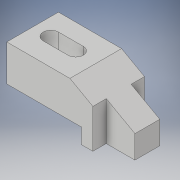
# Autodesk Inventor part: 410571040-T1
Saved by Autodesk Inventor 2017 (Build 210142000, 142)
## iProperties
Part Number: 410571040-T1
Material: 一般
Document SubType Name: Modeling
Designer: user
Density: 1 g/cm^3
Appearance: 預設
Author: user
Autodesk Inventor part; units mm, degrees
ref_plane "YZ Plane" through (0, 0, 0) normal (1, 0, 0) x (0, 1, 0)
ref_plane "XZ Plane" through (0, 0, 0) normal (0, 1, 0) x (-1, 0, 0)
ref_plane "XY Plane" through (0, 0, 0) normal (0, 0, 1) x (1, 0, 0)
sketch "草圖1" plane through (0, 0, 0) normal (0, 0, 1) x (1, 0, 0)
  line L0 (0, 0) -> (0, 38)
  line L1 (0, 38) -> (66, 38)
  line L2 (66, 38) -> (120, 8)
  line L3 (120, 8) -> (120, -16)
  line L4 (120, -16) -> (78, -16)
  line L5 (78, -16) -> (78, 0)
  line L6 (78, 0) -> (0, 0)
  dimension "d0" = 54
  dimension "d1" = 38
  dimension "d2" = 24
  dimension "d3" = 42
  dimension "d4" = 66
  dimension "d5" = 120
  constraints: 14 end point, 4 perpendicular, 1 parallel, 1 vertical
  measures "d0" distance between parallel lines of L4 L1
  measures "d1" distance of L0.start L0.end
  measures "d2" distance of L2.end L3.end
  measures "d3" distance of L3.end L4.end
  measures "d4" distance of L0.end L1.end
  measures "d5" distance between parallel lines of L3 L0
extrude "擠出1" add sketch "草圖1" against normal blind 54
sketch "草圖2" plane through (0, 38, 0) normal (0, 1, 0) x (1, 0, 0)
  arc A0 (18, 36) -> (18, 20) centre (18, 28) ccw
  line L0 (18, 36) -> (44, 36)
  line L1 (18, 20) -> (44, 20)
  arc A1 (44, 20) -> (44, 36) centre (44, 28) ccw
  line L2 (0, 0) -> (66, 0) projected
  line L3 (0, 0) -> (0, 54) projected
  dimension "d8" = 28
  dimension "d9" = 16
  dimension "d10" = 18
  dimension "d11" = 26
  constraints: 4 end point, 4 point on circle, 4 tangent, 2 centre point, 1 horizontal, 1 parallel
  measures "d8" distance from line of A0.centre L2
  measures "d9" distance between parallel lines of L1 L0
  measures "d10" distance from line of L3 A0.centre
  measures "d11" distance of A1.centre A0.centre
extrude "擠出2" cut sketch "草圖2" against normal up to next
sketch "草圖3" plane through (78, -16, 0) normal (0, -1, 0) x (1, 0, 0)
  line L0 (12, -54) -> (12, -40)
  line L1 (12, -40) -> (42, -40)
  line L2 (42, -40) -> (42, -54)
  line L3 (42, -54) -> (12, -54)
  line L4 (42, 0) -> (42, -54) projected
  line L5 (42, -27) -> (-15.5842, -27)
  line L6 (12, 0) -> (12, -14)
  line L7 (12, -14) -> (42, -14)
  line L8 (42, -14) -> (42, 0)
  line L9 (42, 0) -> (12, 0)
  line L10 (42, -54) -> (42, 0)
  point P0 (-78, 0)
  point P1 (0, 0)
  point P2 (0, -54)
  point P3 (0, 0)
  dimension "d18" = 30
  dimension "d19" = 14
  constraints: 20 end point, 6 symmetric about line, 3 perpendicular, 1 horizontal, 1 midpoint, 1 vertical
  measures "d18" distance of L2.end L0.start
  measures "d19" distance of L1.end L2.end
extrude "擠出3" cut sketch "草圖3" against normal up to next
